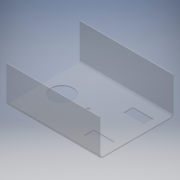
# Autodesk Inventor part: Part2
Saved by Autodesk Inventor 2019 (Build 230136000, 136)
## iProperties
Created: 2019-08-08
Part Number: Part2
Material: PMMA Plastic
Document SubType Name: Modeling
Designer: daozhou.cen
Density: 1.188 g/cm^3
Appearance: Polycarbonate - Clear
Author: daozhou.cen
Autodesk Inventor part; units mm, degrees
ref_plane "YZ Plane" through (0, 0, 0) normal (1, 0, 0) x (0, 1, 0)
ref_plane "XY Plane" through (0, 0, 0) normal (0, 0, 1) x (1, 0, 0)
sketch "Sketch1" plane through (0, 0, 0) normal (1, 0, 0) x (0, 1, 0)
  line L0 (50, -100) -> (-50, -100) construction
  line L1 (-50, -100) -> (-50, 100) construction
  line L2 (-50, 100) -> (50, 100) construction
  line L3 (50, 100) -> (50, -100) construction
  line L4 (50, -100) -> (-50, 100) construction
  line L5 (-50, -100) -> (50, 100) construction
  line L6 (50, 100) -> (-40, 100)
  arc A0 (-40, 100) -> (-50, 90) centre (-40, 90) ccw
  line L7 (50, -100) -> (-40, -100)
  arc A1 (-50, -90) -> (-40, -100) centre (-40, -90) ccw
  line L8 (-50, -90) -> (-50, 90)
  point P0 (0, 0)
  dimension "d0" = 100
  dimension "d1" = 200
  dimension "d2" = 90
  dimension "d3" = 90
  constraints: 18 end point, 4 point on circle, 4 point on line, 4 tangent, 2 centre point, 2 midpoint, 2 parallel, 1 collinear, 1 horizontal, 1 perpendicular
  measures "d0" distance of L1.end L2.end
  measures "d1" distance of L0.end L1.end
  measures "d2" distance of L2.end L6.end
  measures "d3" distance of L0.start L7.end
ref_plane "Work Plane1" through (0, 50, 100) normal (0, 1, 0) x (-1, 0, 0)
sketch "Sketch2" plane through (0, 50, 100) normal (0, 1, 0) x (-1, 0, 0)
  line L0 (56, 0) -> (-194, 0)
  line L1 (-194, 0) -> (-194, -3)
  line L2 (-194, -3) -> (56, -3)
  line L3 (56, -3) -> (56, 0)
  point P0 (0, -100)
  dimension "d4" = 250
  dimension "d5" = 3
  constraints: 8 end point, 2 parallel, 1 horizontal, 1 perpendicular
  measures "d4" distance of L2.end L1.end
  measures "d5" distance of L1.end L0.end
sweep "Sweep1" add profiles "Sketch2" path "Sketch1"
sketch "Sketch3" plane through (-56, -47, 90) normal (0, 1, 0) x (1, 0, 0)
  circle A0 centre (50, 90) radius 30
  line L0 (175, 25) -> (230, 25)
  line L1 (230, 25) -> (230, 50)
  line L2 (230, 50) -> (175, 50)
  line L3 (175, 50) -> (175, 25)
  line L4 (250, 0) -> (250, 180) projected
  line L5 (0, 0) -> (250, 0) projected
  line L6 (56, 90) -> (50, 90) construction
  line L7 (50, 90) -> (250, 90) construction
  line L8 (175, 155) -> (230, 155)
  line L9 (230, 155) -> (230, 130)
  line L10 (230, 130) -> (175, 130)
  line L11 (175, 130) -> (175, 155)
  line L12 (0, 0) -> (0, 180) projected
  circle A1 centre (120, 90) radius 5
  dimension "d8" = 60
  dimension "d10" = 55
  dimension "d11" = 25
  dimension "d12" = 20
  dimension "d13" = 25
  dimension "d25" = 50
  dimension "d26" = 10
  dimension "d27" = 120
  constraints: 20 end point, 4 symmetric about line, 2 centre point, 2 horizontal, 2 parallel, 1 midpoint, 1 perpendicular, 1 point on line
  measures "d8" diameter of A0
  measures "d10" distance of L2.end L1.end
  measures "d11" distance of L1.end L0.end
  measures "d12" distance between parallel lines of L1 L4
  measures "d13" distance between parallel lines of L0 L5
  measures "d25" distance from line of L6.end L12
  measures "d26" diameter of A1
  measures "d27" distance from line of A1.centre L12
extrude "Extrusion1" cut sketch "Sketch3" against normal through all
sketch "Sketch4" plane through (-56, 50, 100) normal (0, 0, 1) x (1, 0, 0)
  line L0 (0, 0) -> (0, -90) projected
  line L1 (250, -90) -> (0, -90) projected
  point P0 (56, -50)
  point P1 (50, -80)
  dimension "d16" = 50
  dimension "d17" = 10
  constraints: 1 other
  measures "d17" distance from line of L1 point (50, -80)
hole "Hole1" at (-6, -30, 100) direction (0, 0, -1) diameter 3 end through all
equation "\"d3\" = d2"
equation "\"d16\" = d9"
equation "\"d9\" = 50"
body "Solid1"
